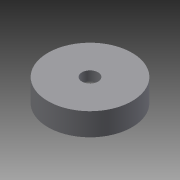
# Autodesk Inventor part: HubCover
Saved by Autodesk Inventor 2014 SP1 (Build 180222100, 222)
## iProperties
Created: 2017-01-21
Part Number: HubCover
Material: Generic
Document SubType Name: Modeling
Designer: danielsikar
Density: 1 g/cm^3
Appearance: Default
Author: danielsikar
Autodesk Inventor part; units mm, degrees
ref_plane "YZ Plane" through (0, 0, 0) normal (1, 0, 0) x (0, 1, 0)
ref_plane "XZ Plane" through (0, 0, 0) normal (0, 1, 0) x (-1, 0, 0)
ref_plane "XY Plane" through (0, 0, 0) normal (0, 0, 1) x (1, 0, 0)
sketch "Sketch1" plane through (0, 0, 0) normal (0, 0, 1) x (1, 0, 0)
  circle A0 centre (0, 0) radius 10.75 projected
  point P0 (0, 0)
extrude "Extrusion1" add sketch "Sketch1" along normal blind 3
sketch "Sketch2" plane through (0, 0, 3) normal (0, 0, 1) x (1, 0, 0)
  circle A0 centre (0, 0) radius 10.75 projected
  circle A1 centre (0, 0) radius 2.5
  dimension "d2" = 5
  constraints: 1 centre point, 1 coincident
  measures "d2" diameter of A1
extrude "Extrusion2" cut sketch "Sketch2" against normal blind 3 contours A1
sketch "Sketch3" plane through (0, 0, 0) normal (0, 0, -1) x (-1, 0, 0)
  circle A0 centre (0, 0) radius 10.75 projected
  circle A1 centre (0, 0) radius 13
  dimension "d5" = 26
  constraints: 1 centre point, 1 coincident
  measures "d5" diameter of A1
extrude "Extrusion3" add sketch "Sketch3" against normal up to surface (3 mm away)
sketch "Sketch4" plane through (0, 0, 0) normal (0, 0, -1) x (-1, 0, 0)
  circle A0 centre (0, 0) radius 13 projected
  circle A1 centre (0, 0) radius 2.5 projected
  circle A2 centre (0, 0) radius 11
  dimension "d8" = 22
  constraints: 1 centre point, 1 coincident
  measures "d8" diameter of A2
extrude "Extrusion4" add sketch "Sketch4" along normal blind 3 contours A0
body "Solid1"
